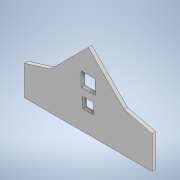
# Autodesk Inventor part: backOfHouseForSiding
Saved by Autodesk Inventor 2020.1 (Build 241239000, 239)
## iProperties
Created: 2019-08-10
Part Number: backOfHouseForSiding
Material: Generic
Document SubType Name: Modeling
Designer: steele
Mass: 1.32952e+07 g
Surface Area: 991051 cm^2
Volume: 1.32952e+07 cm^3
Density: 1 g/cm^3
Appearance: Default
Author: steele
Autodesk Inventor part; units mm, degrees
ref_plane "YZ Plane" through (0, 0, 0) normal (1, 0, 0) x (0, 1, 0)
ref_plane "XZ Plane" through (0, 0, 0) normal (0, 1, 0) x (-1, 0, 0)
ref_plane "XY Plane" through (0, 0, 0) normal (0, 0, 1) x (1, 0, 0)
sketch "Sketch1" plane through (0, 0, 0) normal (0, 0, 1) x (1, 0, 0)
  line L0 (0, 0) -> (5537.2, 0)
  line L1 (0, 0) -> (-5537.2, 0)
  line L2 (-5537.2, 0) -> (-4317.3707, 0)
  line L3 (-5537.2, 0) -> (-5537.2, 2590.8)
  line L4 (-5537.2, 2590.8) -> (-3251.2, 3302)
  line L5 (-3251.2, 3302) -> (0, 6553.2)
  line L6 (0, 0) -> (0, 6553.2) construction
  line L7 (-3251.2, 3302) -> (-3251.2, 0) construction
  line L8 (0, 6553.2) -> (3098.8, 3454.4)
  line L9 (5537.2, 0) -> (5537.2, 2844.8)
  line L10 (5537.2, 2844.8) -> (3098.8, 3454.4)
  line L11 (3098.8, 3454.4) -> (3098.8, 0) construction
  line L12 (-457.2, 1734.6619) -> (457.2, 1734.6619)
  line L13 (457.2, 1734.6619) -> (457.2, 2649.0619)
  line L14 (457.2, 2649.0619) -> (-457.2, 2649.0619)
  line L15 (-457.2, 2649.0619) -> (-457.2, 1734.6619)
  line L16 (-457.2, 1734.6619) -> (457.2, 2649.0619) construction
  line L17 (457.2, 1734.6619) -> (-457.2, 2649.0619) construction
  line L18 (-609.6, 3277.1011) -> (609.6, 3277.1011)
  line L19 (609.6, 3277.1011) -> (609.6, 4496.3011)
  line L20 (609.6, 4496.3011) -> (-609.6, 4496.3011)
  line L21 (-609.6, 4496.3011) -> (-609.6, 3277.1011)
  line L22 (-609.6, 3277.1011) -> (609.6, 4496.3011) construction
  line L23 (609.6, 3277.1011) -> (-609.6, 4496.3011) construction
  point P0 (0, 2191.8619)
  point P1 (0, 3886.7011)
  dimension "d0" = 5537.2
  dimension "d1" = 5537.2
  dimension "d2" = 2590.8
  dimension "d3" = 6553.2
  dimension "d4" = 45
  dimension "d5" = 3302
  dimension "d6" = 3454.4
  dimension "d7" = 45
  dimension "d8" = 914.4
  dimension "d9" = 914.4
  dimension "d10" = 1219.2
  dimension "d11" = 1219.2
  dimension "d14" = 2844.8
  dimension "d15" = 2394.0763
  dimension "d16" = 4597.8911
  dimension "d17" = 4382.365
  dimension "d18" = 2513.4452
  constraints: 48 end point, 6 perpendicular, 6 point on line, 4 midpoint, 4 parallel, 3 vertical, 2 horizontal
  measures "d0" distance of L0.start L0.end
  measures "d1" distance of L0.start L1.end
  measures "d2" distance of L1.end L3.end
  measures "d3" distance of L0.start L6.end
  measures "d4" angle of L5 L6
  measures "d5" distance of L4.end L7.end
  measures "d6" distance of L8.end L11.end
  measures "d7" angle of L6 L8
  measures "d8" distance of L12.start L12.end
  measures "d9" distance of L13.end L12.end
  measures "d10" distance of L18.start L18.end
  measures "d11" distance of L19.end L18.end
  measures "d14" distance of L0.end L9.end
  measures "d15" distance of L4.end L3.end
  measures "d16" distance of L5.end L4.end
  measures "d17" distance of L8.end L6.end
  measures "d18" distance of L9.end L8.end
extrude "Extrusion1" add sketch "Sketch1" against normal blind 304.8
body "Solid1"
